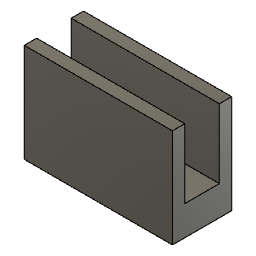
Servo Motor Lock piece v3 (Autodesk Fusion 360 design; units mm, degrees)
Autodesk Fusion 360 part; units mm, degrees
box "BoxPrimitive1" add length 10 width 6 height 15 placed x (0, 1, 0) y (0, 0, 1) z (1, 0, 0) at (0, 0, 0)
sketch "Sketch3" plane through (0, 0, 0) normal (-1, 0, 0) x (0, 0, 1)
  line L0 (6, 10) -> (0, 10)
  line L1 (0, 10) -> (0, 0)
  line L2 (0, 0) -> (6, 0)
  line L3 (6, 0) -> (6, 10)
  line L4 (3, 10) -> (3, 6.5) construction
  line L5 (4.75, 10) -> (1.25, 10)
  line L6 (1.25, 10) -> (1.25, 3)
  line L7 (1.25, 3) -> (4.75, 3)
  line L8 (4.75, 3) -> (4.75, 10)
  line L9 (4.75, 10) -> (1.25, 3) construction
  line L10 (1.25, 10) -> (4.75, 3) construction
  point P0 (3, 6.5)
  dimension "d11" = 3.5
  dimension "d12" = 3.5
  dimension "d13" = 7
  constraint midpoint L0 L4.start
  constraint perpendicular L0 L4
  constraint horizontal L5
  constraint perpendicular L5 L6
  constraint parallel L5 L7
  constraint parallel L6 L8
  constraint coincident L9 P0
  constraint coincident L10 P0
  constraint coincident P0 L4.end
  measures "d11" distance of L4.start P0
  measures "d12" distance of L6.end L7.end
  measures "d13" distance of L5.end L6.end
extrude "Extrude1" cut sketch "Sketch3" against normal blind 15 contours L0 L5 L6 L7 L8
equation "Hole = 3.5 mm"
equation "Width = 6 mm"
equation "Length = 15 mm"
equation "d4 = Height"
equation "d5 = Width"
equation "d6 = Length"
equation "Height = 10 mm"
equation "HHole = 7 mm"
equation "d11 = HHole / 2"
equation "d12 = Hole"
equation "d13 = HHole"
equation "d14 = -Length"
